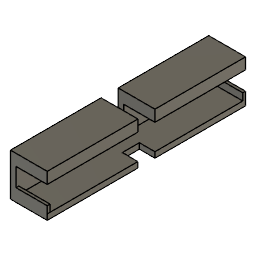
motorHolder (Autodesk Fusion 360 design; units mm, degrees)
part number: 2026-04-07-23-47-39-558
Autodesk Fusion 360 part; units mm, degrees
note: some values were not read from the file. Chosen so that the rebuilt part matches the saved one: which face or edge a step refers to; that a step has no effect.
sketch "Sketch1" plane through (0, 0, 0) normal (0, 1, 0) x (1, 0, 0)
  line L0 (0, 0) -> (11, 0)
  line L1 (11, 0) -> (11, 9)
  line L2 (11, 9) -> (0, 9)
  line L3 (0, 9) -> (0, 0)
  line L4 (11, 20) -> (11, 0)
  line L5 (11, 20) -> (-11, 20)
  line L6 (-11, 20) -> (-11, 0)
  line L7 (-11, 0) -> (0, 0)
  line L8 (0, 9) -> (0, 11)
  line L9 (0, 11) -> (11, 11)
  line L10 (13, 11) -> (13, -2)
  line L11 (13, -2) -> (-1, -2)
  line L12 (-1, -2) -> (-2, -2)
  line L13 (-2, -2) -> (-2, 11)
  line L14 (-2, 11) -> (0, 11)
  line L15 (11, 11) -> (13, 11)
  dimension "d2" = 9
  dimension "d7" = 20
  constraint coincident L0.start L3.end
  constraint horizontal L0
  constraint perpendicular L0 L1
  constraint perpendicular L1 L2
  constraint perpendicular L0 L3
  constraint perpendicular L4 L5
  constraint perpendicular L3 L7
  constraint perpendicular L2 L8
  constraint coincident L4 L9.end
  constraint perpendicular L4 L9
  constraint perpendicular L9 L10
  constraint perpendicular L10 L11
  constraint perpendicular L3 L12
  constraint perpendicular L12 L13
  constraint perpendicular L8 L14
  constraint perpendicular L4 L15
  measures "d2" distance of L0.end L1.end
  measures "d7" distance of L5.end L6.end
extrude "Extrude1" add sketch "Sketch1" along normal blind 70 thin wall 2 inside contours L0 L1 L2 L3 L4 | L3 L7 L8 L13 L14 | L0 L1 L4 L7 L10 L11 L12 L13 L15 | L2 L4 L8 L9
extrude "Extrude2" cut 1 faces at (13, 23.3333, -6.6667) along direction (-1, 0, 0) blind 2
sketch "Sketch2" plane through (0, 0, -9) normal (0, 0, 1) x (-1, 0, 0)
  line L0 (0, 0) -> (-11, 0)
  line L1 (-11, 0) -> (-11, -70)
  line L2 (-11, -70) -> (0, -70)
  line L3 (0, -70) -> (0, 0)
  line L4 (0, 0) -> (0, -1)
  line L5 (-11, -1) -> (-11, 0)
  line L6 (0, 0) -> (0, -1)
  line L7 (-11, -1) -> (0, -1)
  line L8 (0, 0) -> (-11, 0)
  constraint coincident L0.start L3.end
  constraint coincident L3 L4.end
  constraint coincident L1 L5.start
  constraint coincident L0.end L1.start
  constraint perpendicular L6 L7
extrude "Extrude3" add sketch "Sketch2" along normal blind 2.5 contours L0 L1 L3 L4 L5 L6 L7 L8
sketch "Sketch3" plane through (0, 0, -9) normal (0, 0, 1) x (-1, 0, 0)
  line L0 (0, -1) -> (-11, -1)
  line L1 (-11, -1) -> (-11, -70)
  line L2 (-11, -70) -> (0, -70)
  line L3 (0, -70) -> (0, -1)
  line L4 (-11, -70) -> (-11, -69)
  line L5 (0, -69) -> (0, -70)
  line L6 (-11, -69) -> (0, -69)
  line L7 (0, -70) -> (-11, -70)
  constraint coincident L1.end L2.start
  constraint coincident L1 L4.end
  constraint coincident L3 L5.start
  constraint coincident L2.end L3.start
  constraint horizontal L6
extrude "Extrude4" add sketch "Sketch3" along normal blind 2.5 contours L1 L2 L3 L4 L5 L6 L7
sketch "Sketch4" plane through (0, 0, 2) normal (0, 0, 1) x (-1, 0, 0)
  line L0 (-11, 0) -> (-11, -70)
  line L1 (-11, -70) -> (2, -70)
  line L2 (2, -70) -> (2, 0)
  line L3 (2, 0) -> (-11, 0)
  line L4 (-11, 0) -> (-11, -26)
  line L5 (-11, -70) -> (-11, -44)
  line L6 (-11, -44) -> (2, -44)
  line L7 (-11, -26) -> (-10, -26)
  line L8 (-10, -26) -> (2, -26)
  line L9 (2, -44) -> (-11, -44)
  line L10 (-11, -26) -> (-11, -44)
  dimension "d18" = 26
  constraint coincident L0.start L3.end
  constraint perpendicular L3 L4
  constraint coincident L0.end L1.start
  constraint coincident L0 L5.end
  constraint coincident L2 L6.end
  constraint perpendicular L2 L6
  constraint perpendicular L0 L7
  constraint coincident L2 L8.end
  constraint perpendicular L2 L8
  measures "d18" distance of L0.start L4.end
extrude "Extrude5" cut sketch "Sketch4" against normal blind 11 contours L0 L2 L6 L7 L8 L9 L10
extrude "Extrude6" add 1 faces at (3, 26, 1.3333) along direction (0, 1, 0) blind 2
sketch "Sketch5" plane through (0, 0, 2) normal (0, 0, 1) x (-1, 0, 0)
  line L0 (2, -28) -> (2, 0)
  line L1 (2, 0) -> (-11, 0)
  line L2 (-11, 0) -> (-11, -28)
  line L3 (-11, -28) -> (2, -28)
  line L4 (-11, -28) -> (-11, -26)
  line L5 (2, -26) -> (-11, -26)
  line L6 (-11, -27) -> (0, -27)
  line L7 (0, -27) -> (0, -26)
  constraint coincident L2.end L3.start
  constraint coincident L2 L4.end
  constraint coincident L0 L5.start
  constraint perpendicular L4 L5
  constraint midpoint L4 L6.start
  constraint perpendicular L2 L6
  constraint coincident L5 L7.end
  constraint perpendicular L5 L7
extrude "Extrude7" cut sketch "Sketch5" against normal blind 3 contours L2 L4 L5 L6 L7
extrude "Extrude8" add 1 faces at (3, 8.6667, 2) along direction (0, 0, 1) blind 2
extrude "Extrude9" add 1 faces at (2.3333, 61.3333, 2) along direction (0, 0, 1) blind 2
sketch "Sketch6" plane through (0, 0, 0) normal (1, 0, 0) x (0, 1, 0)
  line L0 (26, 0) -> (0, 0)
  line L1 (0, 0) -> (0, -6.5)
  line L2 (0, -6.5) -> (1, -6.5)
  line L3 (1, -6.5) -> (1, -9)
  line L4 (1, -9) -> (28, -9)
  line L5 (28, -9) -> (28, 0)
  line L6 (28, 0) -> (27, 0)
  line L7 (27, 0) -> (27, 4)
  line L8 (27, 4) -> (26, 4)
  line L9 (26, 4) -> (26, 0)
  line L10 (27, 2) -> (26, 2)
  line L11 (26, 4) -> (27, 4)
  constraint midpoint L7 L10.start
  constraint midpoint L9 L10.end
  constraint coincident L8.end L9.start
  constraint coincident L7.end L8.start
extrude "Extrude10" add sketch "Sketch6" along normal blind 11 contours L7 L8 L9 L10 L11
sketch "Sketch7" plane through (0, 0, 0) normal (1, 0, 0) x (0, 1, 0)
  line L0 (27, 2) -> (26, 2)
  line L1 (26, 2) -> (26, 0)
  line L2 (26, 0) -> (0, 0)
  line L3 (0, 0) -> (0, -6.5)
  line L4 (0, -6.5) -> (1, -6.5)
  line L5 (1, -6.5) -> (1, -9)
  line L6 (1, -9) -> (28, -9)
  line L7 (28, -9) -> (28, 0)
  line L8 (28, 0) -> (27, 0)
  line L9 (27, 0) -> (27, 2)
  line L10 (26, 0) -> (27, 0)
  constraint coincident L1.end L2.start
  constraint coincident L8.end L9.start
extrude "Extrude11" add sketch "Sketch7" along normal blind 11 contours L0 L1 L9 L10
sketch "Sketch8" plane through (11, 0, 0) normal (1, 0, 0) x (0, 1, 0)
  line L0 (0, 0) -> (28, 0)
  line L1 (28, 0) -> (28, 4)
  line L2 (28, 4) -> (0, 4)
  line L3 (0, 4) -> (0, 0)
extrude "Extrude12" add 1 faces at (3, 44, 2.6667) along direction (0, -1, 0) blind 2
extrude "Extrude13" add 1 faces at (3, 42, 2.6667) along direction (0, -1, 0) blind 2
extrude "Extrude14" add 1 faces at (3, 28, 2.6667) along direction (0, 1, 0) blind 2
extrude "Extrude15" [no effect]
extrude "Extrude16" add 1 faces at (3, 30, 2.6667) along direction (0, 1, 0) blind 2
extrude "Extrude17" add 1 faces at (3, 40, 2.6667) along direction (0, -1, 0) blind 2
sketch "Sketch9" plane through (0, 0, 4) normal (0, 0, 1) x (-1, 0, 0)
  line L0 (-11, -38) -> (-11, -70)
  line L1 (-11, -70) -> (2, -70)
  line L2 (2, -70) -> (2, -38)
  line L3 (2, -38) -> (-11, -38)
extrude "Extrude18" cut 1 faces at (3, 38, 2.6667) along direction (0, 1, 0) blind 2
extrude "Extrude19" cut 1 faces at (3, 32, 2.6667) along direction (0, -1, 0) blind 2
extrude "Extrude20" add 1 faces at (3, 30, 2.6667) along direction (0, 1, 0) blind 2
extrude "Extrude21" add 1 faces at (3, 40, 2.6667) along direction (0, -1, 0) blind 2
sketch "Sketch10" plane through (11, 0, 0) normal (1, 0, 0) x (0, 1, 0)
  line L0 (32, 4) -> (0, 4)
  line L1 (0, 4) -> (0, 0)
  line L2 (0, 0) -> (32, 0)
  line L3 (32, 0) -> (32, 4)
  line L4 (32, 0) -> (30, 0)
  line L5 (30, 0) -> (30, 2.5)
  line L6 (30, 2.5) -> (28, 2.5)
  line L7 (28, 2.5) -> (28, 0)
  constraint coincident L2.end L3.start
  constraint coincident L2 L4.end
  constraint perpendicular L4 L5
  constraint perpendicular L5 L6
  constraint coincident L2 L7.end
  constraint perpendicular L2 L7
extrude "Extrude22" cut sketch "Sketch10" against normal blind 20 contours L2 L5 L6 L7
sketch "Sketch11" plane through (11, 0, 0) normal (1, 0, 0) x (0, 1, 0)
  line L0 (38, 0) -> (70, 0)
  line L1 (70, 0) -> (70, 4)
  line L2 (70, 4) -> (38, 4)
  line L3 (38, 4) -> (38, 0)
  line L4 (38, 0) -> (40, 0)
  line L5 (40, 0) -> (40, 2.5)
  line L6 (40, 2.5) -> (42, 2.5)
  line L7 (42, 2.5) -> (42, 0)
  constraint coincident L0.start L3.end
  constraint coincident L0 L4.end
  constraint perpendicular L4 L5
  constraint perpendicular L5 L6
  constraint coincident L0 L7.end
  constraint perpendicular L0 L7
extrude "Extrude23" cut sketch "Sketch11" against normal blind 21 contours L0 L5 L6 L7
extrude "Extrude24" add 1 faces at (3, 30, 1.6667) along direction (0, -1, 0) blind 2
extrude "Extrude25" add 1 faces at (3, 42, 1.6667) along direction (0, -1, 0) blind 2
sketch "Sketch12" plane through (0, 0, -9) normal (0, 0, 1) x (-1, 0, 0)
  line L0 (0, -69) -> (0, -38)
  line L1 (0, -38) -> (2, -38)
  line L2 (2, -38) -> (2, -32)
  line L3 (2, -32) -> (0, -32)
  line L4 (0, -32) -> (0, -1)
  line L5 (0, -1) -> (-11, -1)
  line L6 (-11, -1) -> (-11, -69)
  line L7 (-11, -69) -> (0, -69)
  line L8 (0, -32) -> (-11, -32)
  line L9 (0, -38) -> (-11, -38)
  line L10 (-11, -32) -> (-5.5093, -32)
  line L11 (-5.5, -38) -> (-11, -38)
  line L12 (-11, -32) -> (-5.5093, -32)
  line L13 (-5.5093, -32) -> (-5.5, -38)
  constraint coincident L3.end L4.start
  constraint coincident L6 L8.end
  constraint perpendicular L6 L8
  constraint coincident L0.end L1.start
  constraint coincident L6 L9.end
  constraint perpendicular L6 L9
  constraint midpoint L9 L11.start
extrude "Extrude26" cut sketch "Sketch12" against normal blind 4 contours L6 L8 L9 L10 L11 L12 L13
